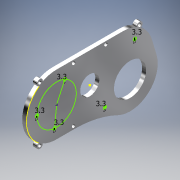
# Autodesk Inventor part: Gearbox Plate 1
Saved by Autodesk Inventor 2019.4 (Build 234330000, 330)
## iProperties
Created: 2019-12-11
Part Number: Gearbox Plate 1
Material: Aluminum 6061
Document SubType Name: Modeling
Designer: admin
Density: 2.7 g/cm^3
Appearance: Aluminum - Flat
Author: admin
Autodesk Inventor part; units mm, degrees
ref_plane "YZ Plane" through (0, 0, 0) normal (1, 0, 0) x (0, 1, 0)
ref_plane "XZ Plane" through (0, 0, 0) normal (0, 1, 0) x (-1, 0, 0)
ref_plane "XY Plane" through (0, 0, 0) normal (0, 0, 1) x (1, 0, 0)
sketch "Sketch1" plane through (0, 0, 0) normal (1, 0, 0) x (0, 1, 0)
  arc A0 (-30, 33.02) -> (30, 33.02) centre (0, 33.02) ccw construction
  arc A1 (30, -33.02) -> (-30, -33.02) centre (0, -33.02) ccw construction
  line L0 (0, 33.02) -> (0, -33.02) construction
  line L1 (30, 33.02) -> (30, -33.02)
  line L2 (-30, -33.02) -> (-30, -17.0216) construction
  arc A2 (30, 33.02) -> (-30, 33.02) centre (0, 33.02) ccw
  arc A3 (-30, -33.02) -> (-29.9675, -34.4159) centre (0, -33.02) ccw
  circle A4 centre (0, 0) radius 9.5
  circle A5 centre (-15, -40.0705) radius 16
  line L3 (0, 0) -> (-15, -40.0705) construction
  arc A6 (0.1521, -63.0196) -> (-30, -17.0216) centre (-15, -40.0705) ccw construction
  arc A7 (-30, -17.0216) -> (0.1521, -63.0196) centre (-15, -40.0705) ccw
  arc A8 (-20.197, -55.2029) -> (0.1521, -63.0196) centre (0, -33.02) ccw construction
  arc A9 (-29.9675, -34.4159) -> (-20.197, -55.2029) centre (0, -33.02) ccw construction
  line L4 (-30, -17.0216) -> (-30, 33.02)
  arc A10 (0.1521, -63.0196) -> (30, -33.02) centre (0, -33.02) ccw
  line L5 (-7.1898, -66.4381) -> (8.5203, -61.7846)
  dimension "d0" = 60
  dimension "d1" = 60
  dimension "d2" = 66.04
  dimension "d3" = 19
  dimension "d10" = 32
  dimension "d12" = 42.786
  dimension "d13" = 15
  dimension "d14" = 55
  constraints: 23 point on circle, 12 end point, 11 centre point, 8 tangent, 3 coincident, 1 midpoint, 1 vertical
  measures "d0" diameter of A0
  measures "d1" diameter of A1
  measures "d2" distance of L0.end L0.start
  measures "d3" diameter of A4
  measures "d10" diameter of A5
  measures "d12" distance of L3.start L3.end
  measures "d13" horizontal distance of L0.end L3.end
  measures "d14" diameter of A6
extrude "Extrusion1" add sketch "Sketch1" along normal blind 4
fillet "Fillet1" radius 100 1 edges at (2, -30, -17.0216)
sketch "Sketch2" plane through (4, 0, 0) normal (1, 0, 0) x (0, 0, -1)
  circle A0 centre (-49.4954, 27.0713) radius 1.65 projected
  circle A1 centre (-49.5731, -26.9286) radius 1.65 projected
  arc A2 (-50.7357, -24.163) -> (-46.5809, -26.7125) centre (-49.5731, -26.9286) ccw projected
  arc A3 (-46.5038, 26.8465) -> (-50.6659, 24.3091) centre (-49.4954, 27.0713) ccw projected
  circle A4 centre (49.5731, 26.9286) radius 1.65 projected
  arc A5 (50.7357, 24.163) -> (46.5809, 26.7125) centre (49.5731, 26.9286) ccw projected
  circle A6 centre (-49.4954, 27.0713) radius 3
  circle A7 centre (-49.5731, -26.9286) radius 3
  circle A8 centre (49.5731, 26.9286) radius 3
  point P0 (0, 0)
  constraints: 3 centre point, 3 coincident, 3 concentric
extrude "Extrusion2" add sketch "Sketch2" against normal up to surface (4 mm away)
sketch "Sketch3" plane through (4, 0, 0) normal (1, 0, 0) x (0, 0, -1)
  circle A0 centre (-15.9811, 27.023) radius 1.65 projected
  circle A1 centre (16.0589, 26.9769) radius 1.65 projected
  circle A2 centre (-16.0589, -26.9769) radius 1.65 projected
  circle A3 centre (15.9811, -27.023) radius 1.65 projected
  point P0 (0, 0)
extrude "Extrusion3" cut sketch "Sketch3" against normal blind 10 contours A0 | A1 | A2
sketch "Sketch4" plane through (4, 0, 0) normal (1, 0, 0) x (0, 0, -1)
  circle A0 centre (-33.02, -22.5) radius 1.65
  circle A1 centre (-55.52, 0) radius 1.65
  circle A2 centre (-33.02, 22.5) radius 1.65
  circle A3 centre (45.02, 17.5) radius 1.65
  circle A4 centre (10.0137, -26) radius 1.65
  arc A5 (-50.6242, 24.2918) -> (-50.7766, -24.1806) centre (-33.02, 0) ccw projected
  circle A6 centre (-33.02, 0) radius 22.5 construction
  line L0 (-33.02, 22.5) -> (-33.02, 0) construction
  line L1 (-33.02, 0) -> (-33.02, -22.5) construction
  line L2 (33.02, 30) -> (-33.02, 30) projected
  arc A7 (61.7846, 8.5203) -> (50.7766, 24.1806) centre (33.02, 0) ccw projected
  line L3 (-33.02, -30) -> (-14.9863, -30) projected
  circle A8 centre (48.0705, -35.855) radius 1.65
  arc A9 (28.1955, -39.8039) -> (66.4381, -7.1898) centre (40.0705, -15) ccw projected
  line L4 (-55.52, 0) -> (-33.02, 0) construction
  point P0 (0, 0)
  dimension "d20" = 3.3
  dimension "d21" = 3.3
  dimension "d22" = 3.3
  dimension "d23" = 3.3
  dimension "d24" = 3.3
  dimension "d25" = 45
  dimension "d26" = 12.5
  dimension "d27" = 12
  dimension "d28" = 4
  dimension "d29" = 25
  dimension "d30" = 3.3
  dimension "d31" = 20.855
  dimension "d32" = 8
  constraints: 7 centre point, 6 end point, 3 point on circle, 1 coincident, 1 collinear, 1 horizontal, 1 vertical
  measures "d20" diameter of A0
  measures "d21" diameter of A1
  measures "d22" diameter of A2
  measures "d23" diameter of A3
  measures "d24" diameter of A4
  measures "d25" diameter of A6
  measures "d26" distance from line of L2 A3.centre
  measures "d27" horizontal distance of A7.centre A3.centre
  measures "d28" distance from line of L3 A4.centre
  measures "d29" horizontal distance of L3.end A4.centre
  measures "d30" diameter of A8
  measures "d31" vertical distance of A9.centre A8.centre
  measures "d32" horizontal distance of A9.centre A8.centre
extrude "Extrusion4" cut sketch "Sketch4" against normal through all
body "Solid1"
